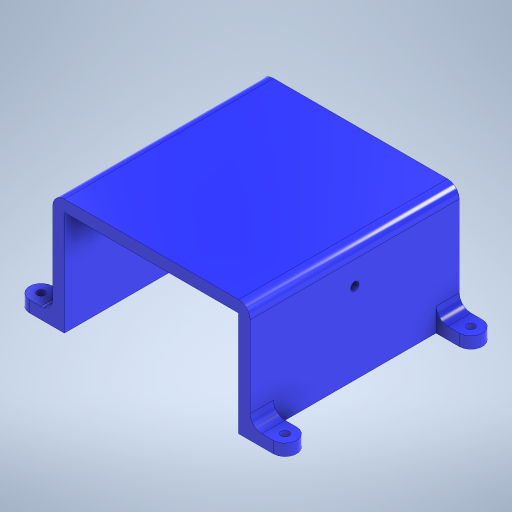
# Autodesk Inventor part: lipobox
Saved by Autodesk Inventor 2023 (Build 270158000, 158)
## iProperties
Created: 2023-04-14
Part Number: lipobox
Material: ABS プラスチック
Document SubType Name: Modeling
Designer: zegi
Density: 1.06 g/cm^3
Appearance: 青 - 壁塗料 - 光沢
Author: zegi
Autodesk Inventor part; units mm, degrees
ref_plane "YZ Plane" through (0, 0, 0) normal (1, 0, 0) x (0, 1, 0)
ref_plane "XZ Plane" through (0, 0, 0) normal (0, 1, 0) x (-1, 0, 0)
sketch "スケッチ1" plane through (0, 0, 0) normal (0, 0, 1) x (1, 0, 0)
  line L0 (0, 50) -> (42.5, 50)
  line L1 (42.5, 50) -> (42.5, 5)
  line L2 (42.5, 5) -> (57.5, 5)
  line L3 (57.5, 5) -> (57.5, 0)
  line L4 (57.5, 0) -> (37.5, 0)
  line L5 (37.5, 0) -> (37.5, 45)
  line L6 (37.5, 45) -> (0, 45)
  line L7 (0, 45) -> (0, 50)
  line L8 (42.5, 5) -> (42.5, 0)
  point P0 (0, 0)
  point P1 (42.5, 27.5)
  point P2 (18.75, 45)
  dimension "d0" = 5
  dimension "d1" = 5
  dimension "d2" = 5
  dimension "d4" = 45
  dimension "d5" = 37.5
  dimension "d6" = 15
  constraints: 18 end point, 8 perpendicular, 2 midpoint, 1 horizontal, 1 horizontal alignment, 1 point on line, 1 vertical alignment
  measures "d0" distance between parallel lines of L0 L6
  measures "d1" distance from line of point (42.5, 27.5) L5
  measures "d2" distance between parallel lines of L4 L2
  measures "d4" distance of point (0, 0) L6.end
  measures "d5" distance of point (0, 0) L4.end
  measures "d6" distance of L8.end L3.end
extrude "押し出し1" add sketch "スケッチ1" along normal blind 45 contours L0 L1 L8 L4 L5 L6 L7
ref_plane "作業平面1" through (0, 0, 40) normal (0, 0, 1) x (1, 0, 0)
extrude "押し出し2" add sketch "スケッチ1" along normal mid plane 10 from surface at 40 contours L2 L3 L4 L8
sketch "スケッチ4" plane through (42.5, 5, 35) normal (0, 1, 0) x (1, 0, 0)
  line L0 (15, -10) -> (15, 0) projected
  line L1 (0, -10) -> (15, -10) projected
  point P0 (-42.5, 35)
  point P1 (10, -5)
  point P2 (15, -5)
  point P3 (7.5, -10)
  dimension "d23" = 5
  constraints: 2 midpoint, 1 horizontal alignment
  measures "d23" distance from line of L0 point (10, -5)
hole "穴1" at (52.5, 5, 40) direction (0, -1, 0) diameter 3.5 end through all
fillet "フィレット1" radius 5 3 edges at (57.5, 2.5, 45) (57.5, 2.5, 35) (42.5, 50, 22.5)
fillet "フィレット2" radius 5 1 edges at (42.5, 5, 40)
mirror "ミラー1" about plane through (21.25, 25, 0) normal (0, 0, -1) of "押し出し1", "フィレット1", "フィレット2", "穴1", "押し出し2"
mirror "ミラー2" about plane through (0, 50, 0) normal (-1, 0, 0) of "押し出し1", "フィレット1", "フィレット2", "穴1", "押し出し2", "ミラー1"
sketch "スケッチ5" plane through (42.5, 10, 45) normal (1, 0, 0) x (0, 0, -1)
  line L0 (90, 35) -> (0, 35) projected
  line L1 (90, 40) -> (0, 40) projected
  point P0 (45, -10)
  point P1 (45, 25)
  point P2 (45, 40)
  dimension "d29" = 10
  constraints: 1 midpoint, 1 vertical alignment
  measures "d29" distance from line of L0 point (45, 25)
hole "穴2" at (42.5, 35, 0) direction (-1, 0, 0) diameter 3.5 end through all
